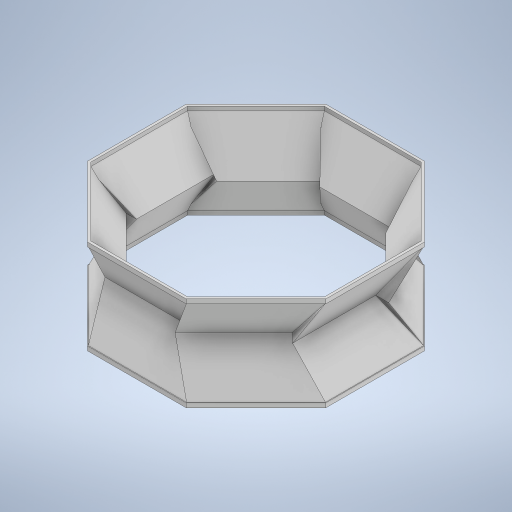
# Autodesk Inventor part: 팔각형 OV-PAM 층 한개
Saved by Autodesk Inventor 2024 (Build 280153000, 153)
## iProperties
Created: 2023-06-16
Part Number: 팔각형 OV-PAM 층 한개
Material: 일반
Document SubType Name: Modeling
Designer: jsw
Density: 1 g/cm^3
Appearance: 기본값
Author: jsw
Autodesk Inventor part; units mm, degrees
ref_plane "YZ Plane" through (0, 0, 0) normal (1, 0, 0) x (0, 1, 0)
sketch "스케치1" plane through (0, 0, 0) normal (0, 1, 0) x (-1, 0, 0)
  line L0 (-32.5919, 13.5) -> (-13.5, 32.5919)
  line L1 (-13.5, 32.5919) -> (13.5, 32.5919)
  line L2 (13.5, 32.5919) -> (32.5919, 13.5)
  line L3 (32.5919, 13.5) -> (32.5919, -13.5)
  line L4 (32.5919, -13.5) -> (13.5, -32.5919)
  line L5 (13.5, -32.5919) -> (-13.5, -32.5919)
  line L6 (-13.5, -32.5919) -> (-32.5919, -13.5)
  line L7 (-32.5919, -13.5) -> (-32.5919, 13.5)
  line L8 (-13.7485, 33.1919) -> (13.7485, 33.1919)
  line L9 (13.7485, 33.1919) -> (33.1919, 13.7485)
  line L10 (33.1919, 13.7485) -> (33.1919, -13.7485)
  line L11 (33.1919, -13.7485) -> (13.7485, -33.1919)
  line L12 (13.7485, -33.1919) -> (-13.7485, -33.1919)
  line L13 (-13.7485, -33.1919) -> (-33.1919, -13.7485)
  line L14 (-33.1919, -13.7485) -> (-33.1919, 13.7485)
  line L15 (-33.1919, 13.7485) -> (-13.7485, 33.1919)
  point P0 (0, 0)
  point P1 (0, 0)
  point P2 (0, 0)
  dimension "d0" = 27
  dimension "d2" = 0.6
  constraints: 32 end point, 2 coincident, 2 horizontal, 34 other
  measures "d0" distance of L0.end L1.end
  measures "d2" distance between parallel lines of L10 L3
extrude "돌출2" add sketch "스케치1" along normal blind 12 contours L0 L1 L2 L3 L4 L5 L6 L7 | L8 L9 L10 L11 L12 L13 L14 L15
ref_plane "작업 평면2" through (33.1919, 0, 13.7485) normal (-0.8660254, -0.5, 0) x (0, 0, -1)
sketch "스케치3" plane through (33.1919, 0, 13.7485) normal (1, 0, 0) x (0, 0, -1)
  line L0 (0, 0) -> (0, 12) projected
  line L1 (0, 12) -> (27.4971, 12) projected
  line L2 (0, 0) -> (27.4971, 0)
  line L3 (27.4971, 0) -> (27.4971, 12)
  line L4 (27.4971, 12) -> (0, 12)
  line L5 (0, 12) -> (0, 0)
  line L6 (0, 12) -> (-7.3047, 12)
  line L7 (-19.4434, 12) -> (0, 12) projected
  line L8 (0, 0) -> (-7.3047, 12)
  line L9 (27.4971, 12) -> (13.7485, 12)
  line L10 (20.9971, 12) -> (27.4971, 0)
  point P0 (13.7485, 0)
  point P1 (20.9971, 12)
  dimension "d17" = 121.33
  dimension "d53" = 6.5
  constraints: 16 end point, 5 midpoint, 2 parallel, 2 point on line, 1 horizontal, 1 perpendicular
  measures "d17" angle of L8 L2
  measures "d53" distance of L1.end L10.start
extrude "돌출4" cut sketch "스케치3" against normal up to surface contours L8 L6 L0 | L0 L1 L10 L2 surface through (33.1919, 0, 13.7485) normal (-0.8660254, -0.5, 0)
pattern_circular "원형 패턴1" count 8 over 360 about axis through (0, -10, 0) along (0, 1, 0) of "돌출4"
mirror "미러5" about plane through (0, 12, 0) normal (0, 1, 0) of "돌출2", "돌출4", "원형 패턴1"
sketch "스케치9" plane through (-13.7485, 24, -33.1919) normal (0, 1, 0) x (1, 0, 0)
  line L0 (46.9404, -46.9404) -> (46.9404, -19.4434) projected
  line L1 (46.9404, -19.4434) -> (27.4971, 0) projected
  line L2 (27.4971, 0) -> (0, 0) projected
  line L3 (0, 0) -> (-19.4434, -19.4434) projected
  line L4 (-19.4434, -19.4434) -> (-19.4434, -46.9404) projected
  line L5 (-19.4434, -46.9404) -> (0, -66.3838) projected
  line L6 (0, -66.3838) -> (27.4971, -66.3838) projected
  line L7 (27.4971, -66.3838) -> (46.9404, -46.9404) projected
  point P0 (13.7485, -33.1919)
extrude "돌출8" add sketch "스케치9" along normal blind 1.2
sketch "스케치10" plane through (0, 0, 0) normal (0, -1, 0) x (1, 0, 0)
  line L0 (33.1919, 13.7485) -> (33.1919, -13.7485) projected
  line L1 (13.7485, 33.1919) -> (33.1919, 13.7485) projected
  line L2 (-13.7485, 33.1919) -> (13.7485, 33.1919) projected
  line L3 (-33.1919, 13.7485) -> (-13.7485, 33.1919) projected
  line L4 (-33.1919, -13.7485) -> (-33.1919, 13.7485) projected
  line L5 (-13.7485, -33.1919) -> (-33.1919, -13.7485) projected
  line L6 (13.7485, -33.1919) -> (-13.7485, -33.1919) projected
  line L7 (33.1919, -13.7485) -> (13.7485, -33.1919) projected
  point P0 (0, 0)
extrude "돌출9" add sketch "스케치10" along normal blind 1.2
shell "쉘6" thickness 0.5 removed faces 2 at (4.5828, 25.2, 11.064) at (4.5828, -1.2, -1.8983)
sketch "스케치12" plane through (-13.7485, 25.2, -33.1919) normal (0, 1, 0) x (1, 0, 0)
  line L0 (46.4404, -19.6505) -> (46.4404, -46.7333) projected
  line L1 (46.4404, -46.7333) -> (27.2899, -65.8838) projected
  line L2 (27.2899, -65.8838) -> (0.2071, -65.8838) projected
  line L3 (0.2071, -65.8838) -> (-18.9434, -46.7333) projected
  line L4 (-18.9434, -46.7333) -> (-18.9434, -19.6505) projected
  line L5 (-18.9434, -19.6505) -> (0.2071, -0.5) projected
  line L6 (0.2071, -0.5) -> (27.2899, -0.5) projected
  line L7 (27.2899, -0.5) -> (46.4404, -19.6505) projected
  line L8 (46.9404, -19.4434) -> (27.4971, 0) projected
  line L9 (27.4971, 0) -> (0, 0) projected
  line L10 (0, 0) -> (-19.4434, -19.4434) projected
  line L11 (-19.4434, -19.4434) -> (-19.4434, -46.9404) projected
  line L12 (-19.4434, -46.9404) -> (0, -66.3838) projected
  line L13 (0, -66.3838) -> (27.4971, -66.3838) projected
  line L14 (27.4971, -66.3838) -> (46.9404, -46.9404) projected
  line L15 (46.9404, -46.9404) -> (46.9404, -19.4434) projected
  line L16 (-0.0828, 0.2) -> (27.5799, 0.2)
  line L17 (27.5799, 0.2) -> (47.1404, -19.3605)
  line L18 (47.1404, -19.3605) -> (47.1404, -47.0233)
  line L19 (47.1404, -47.0233) -> (27.5799, -66.5838)
  line L20 (27.5799, -66.5838) -> (-0.0828, -66.5838)
  line L21 (-0.0828, -66.5838) -> (-19.6434, -47.0233)
  line L22 (-19.6434, -47.0233) -> (-19.6434, -19.3605)
  line L23 (-19.6434, -19.3605) -> (-0.0828, 0.2)
  point P0 (13.7485, -33.1919)
  point P1 (13.7485, -33.1919)
  dimension "d50" = 0.2
  constraints: 16 end point, 1 coincident, 1 horizontal, 17 other
  measures "d50" distance between parallel lines of L9 L16
extrude "돌출10" add sketch "스케치12" against normal blind 1.2 contours L16 L17 L18 L19 L20 L21 L22 L23
ref_plane "작업 평면6" through (-13.7485, 12, -33.1919) normal (0, 1, 0) x (1, 0, 0)
mirror "미러8" about plane through (-13.7485, 12, -33.1919) normal (0, 1, 0) of "돌출10"
